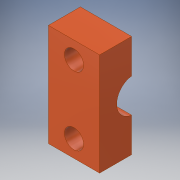
# Autodesk Inventor part: X-axis Rod holder
Saved by Autodesk Inventor 2018 (Build 220112000, 112)
## iProperties
Created: 2013-10-26
Part Number: X-axis Rod holder
Material: ABS Plastic
Document SubType Name: Modeling
Designer: Gabriel Smolnycki
Mass: 1.76778 g
Surface Area: 12.6567 cm^2
Volume: 1.66772 cm^3
Density: 1.06 g/cm^3
Appearance: Smooth - Light Orange
Author: Gabriel Smolnycki
Sending System: SolidWorks 2017
Last Author: Gabriel Smolnycki
Last Saved: 2017-09-14
Autodesk Inventor part; units mm, degrees
ref_plane "YZ Plane" through (0, 0, 0) normal (1, 0, 0) x (0, 1, 0)
ref_plane "XZ Plane" through (0, 0, 0) normal (0, 1, 0) x (-1, 0, 0)
ref_plane "XY Plane" through (0, 0, 0) normal (0, 0, 1) x (1, 0, 0)
sketch "Sketch1" plane through (0, 0, 0) normal (1, 0, 0) x (0, 1, 0)
  arc A0 (3.9686, -7.5) -> (-3.9686, -7.5) centre (0, -8) ccw
  line L0 (3.9686, -7.5) -> (12, -7.5)
  line L1 (-12, -7.5) -> (-3.9686, -7.5)
  line L2 (-12, 0) -> (-12, -7.5)
  line L3 (12, -7.5) -> (12, 0)
  line L4 (12, 0) -> (-12, 0)
  constraints: 10 end point, 3 horizontal, 2 collinear, 2 point on circle, 2 vertical, 1 centre point
extrude "Extrusion1" add sketch "Sketch1" along normal blind 12
hole "Hole2" at (6, -8, 0) direction (0, 0, -1) diameter 4.5 depth 7.5
sketch "Sketch2" plane through (0, 0, 0) normal (0, 0, 1) x (1, 0, 0)
  point P0 (6, -8)
hole "Hole1" at (6, 8, 0) direction (0, 0, -1) diameter 4.5 depth 7.5
sketch "Sketch3" plane through (0, 0, 0) normal (0, 0, 1) x (1, 0, 0)
  point P0 (6, 8)
body "Solid3"
